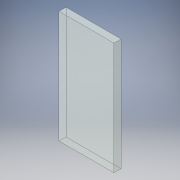
# Autodesk Inventor part: glass slide
Saved by Autodesk Inventor 2019 (Build 230136000, 136)
## iProperties
Created: 2019-03-15
Part Number: glass slide
Material: Glass
Document SubType Name: Modeling
Designer: Saumya
Density: 2.18 g/cm^3
Appearance: Clear
Author: Saumya
Autodesk Inventor part; units mm, degrees
ref_plane "YZ Plane" through (0, 0, 0) normal (1, 0, 0) x (0, 1, 0)
ref_plane "XZ Plane" through (0, 0, 0) normal (0, 1, 0) x (-1, 0, 0)
ref_plane "XY Plane" through (0, 0, 0) normal (0, 0, 1) x (1, 0, 0)
sketch "Sketch1" plane through (0, 0, 0) normal (0, 0, 1) x (1, 0, 0)
  line L0 (16.823, 33.9245) -> (26.7544, 33.9245)
  line L1 (26.7544, 33.9245) -> (26.7544, 13.6441)
  line L2 (26.7544, 13.6441) -> (16.823, 13.6441)
  line L3 (16.823, 13.6441) -> (16.823, 33.9245)
  point P0 (0, 0)
  dimension "d0" = 9.9314
  constraints: 8 end point, 2 parallel, 1 horizontal, 1 perpendicular
  measures "d0" distance of L0.start L0.end
extrude "Extrusion1" add sketch "Sketch1" along normal blind 1.27
body "Solid1"
